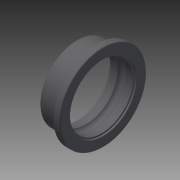
# Autodesk Inventor part: MF74ZZ Outer Ring
Saved by Autodesk Inventor 2014 SP2 (Build 180246200, 246)
## iProperties
Created: 2019-11-12
Part Number: MF74ZZ Outer Ring
Material: Generic
Catalog Web Link: www.cadenas.de
Description: shielded_type_zz_zzs_OR-
Vendor: NSK_RB
Document SubType Name: Modeling
Designer: psadmin
Manufacturer: NSK_RB
Mass: 0.031075 g
Surface Area: 1.54949 cm^2
Volume: 0.031075 cm^3
Density: 1 g/cm^3
Appearance: PSOLRGB-128-128-128
Category: PARTsolutions
Company: NSK_RB
Title: MF74ZZ Outer Ring
Author: Cadenas PARTsolutions
PSOL_IDENT_0: {$CADENAS_DATA\23d-libs\nsk_rb\roller_bearings\deep_groove_bb\exstra_small_miniatur_bb\metric_design
PSOL_IDENT_1: _with_flange\shielded_type_zz_zzs_or1.prj},192 {VTYP=3D},{NB=MF74ZZ Outer Ring},{LINA=MF74ZZ Outer R
PSOL_IDENT_2: ing},{NN=shielded_type_zz_zzs_OR},{DATE=16.01.2019 01:41:14},{GEOMDATE=04.01.2008 00:00:00},{VERSION=
PSOL_IDENT_3: },{LINEID=290},{WBVAR=},{WBNUMERIC=}  {NB=MF74ZZ Outer Ring},{LINA=MF74ZZ Outer Ring},{KT=DUMMY},{ID
PSOL_IDENT_4: NR=},{STAN=},{ORDER=MF74ZZ},{SD=4.0},{X=4.0},{D=7},{DD=7},{DD1=0.0},{D2=8.2},{DD2=8.2},{B=0.0},{B1=2
PSOL_IDENT_5: .5},{CC1=0.0},{C2=0.6},{CC2=0.6},{R=0.00},{R1=0.10},{DI1=4.80},{DI2=4.80},{SDE1=6.00},{SDE2=6.30},{C
PSOL_IDENT_6: R1=255},{COR1=107},{CR2=26},{COR2=11.0},{LG=60000},{LO=67000},{DA=0.0},{DB=4.8},{RA=0.00},{RB=0.10},
PSOL_IDENT_7: {MASS=0.35},{SC=1}
NN: shielded_type_zz_zzs_OR
NB: MF74ZZ Outer Ring
NBSYN: $ORDER. Outer Ring
LINA: MF74ZZ Outer Ring
ORDER: MF74ZZ
SD: 4
X: 4
D: 7
DD: 7
DD1: 0
D2: 8.2
DD2: 8.2
B: 0
B1: 2.5
CC1: 0
C2: 0.6
CC2: 0.6
R: 0
R1: 0.1
DI1: 4.8
DI2: 4.8
SDE1: 6
SDE2: 6.3
CR1: 255
COR1: 107
CR2: 26
COR2: 11
LG: 60000
LO: 67000
DA: 0
DB: 4.8
RA: 0
RB: 0.1
MASS: 0.35
SC: 1
SUPPLIER: NSK_RB
ARTICLENO: MF74ZZ Outer Ring
BOMINFO: MF74ZZ Outer Ring
CREATOR: CADENAS GmbH
Autodesk Inventor part; units mm, degrees
sketch "Sketch_1" plane through (0, 0, 0) normal (0, 0, 1) x (1, 0, 0)
  line L0 (2.5, 0) -> (0, 0)
  line L1 (0, 3.15) -> (0.1562, 3.15)
  line L2 (0.1562, 3.15) -> (0.1562, 3)
  line L3 (0.1562, 3) -> (0.8758, 3)
  arc A0 (1.6242, 3) -> (0.8758, 3) centre (1.25, 2.75) ccw
  line L4 (1.6242, 3) -> (2.3438, 3)
  line L5 (2.3438, 3) -> (2.3438, 3.15)
  line L6 (2.3438, 3.15) -> (2.5, 3.15)
  line L7 (2.5, 3.15) -> (2.5, 4)
  arc A1 (2.5, 4) -> (2.4, 4.1) centre (2.4, 4) ccw
  line L8 (2.4, 4.1) -> (1.9, 4.1)
  line L9 (1.9, 4.1) -> (1.9, 3.5)
  line L10 (1.9, 3.5) -> (0.1, 3.5)
  arc A2 (0.1, 3.5) -> (0, 3.4) centre (0.1, 3.4) ccw
  line L11 (0, 3.4) -> (0, 3.15)
  constraints: 24 end point, 6 point on circle, 3 centre point
revolve "Revolution1" add sketch "Sketch_1" angle 360 about axis through (2.5, 0, 0) along (1, 0, 0)
ref_plane "ip_st_1_XY" through (0, 0, 0) normal (1, 0, 0) x (0, 0, -1)
ref_plane "ip_st_1_YZ" through (0, 0, 0) normal (0, 0, -1) x (0, 1, 0)
ref_plane "ip_st_1_ZX" through (0, 0, 0) normal (0, 1, 0) x (1, 0, 0)
ref_plane "ip_st_2_XY" through (2.3438, 0, 0) normal (-1, 0, 0) x (0, 0, -1)
ref_plane "ip_st_2_YZ" through (2.3438, 0, 0) normal (0, 0, -1) x (0, -1, 0)
ref_plane "ip_st_2_ZX" through (2.3438, 0, 0) normal (0, -1, 0) x (-1, 0, 0)
body "Solid1"
